Autodesk Fusion 360 part; units mm, degrees
note: some values were not read from the file. Chosen so that the rebuilt part matches the saved one: which bodies a step acts on; which face or edge a step refers to. Set by a fixed rule: which sketch regions a step uses.
(part 3 of 3)
sketch "Sketch30" plane through (0, 0, -52.6306) normal (0, 0, -1) x (1, 0, 0)
  line L0 (227.3311, -240.0788) -> (240.3311, -240.0788)
  line L1 (240.3311, -240.0788) -> (240.3311, -235.0788)
  line L2 (240.3311, -235.0788) -> (227.3311, -235.0788)
  line L3 (227.3311, -235.0788) -> (227.3311, -240.0788)
  line L4 (285, -250) -> (219.7748, -250)
  line L5 (219.7748, -250) -> (219.7748, 15.8116)
  line L6 (219.7748, 15.8116) -> (285, 15.8116)
  line L7 (285, 15.8116) -> (285, -250)
  line L8 (213.7748, -256) -> (213.7748, 21.8116)
  line L9 (213.7748, 21.8116) -> (291, 21.8116)
  line L10 (291, 21.8116) -> (291, -256)
  line L11 (291, -256) -> (213.7748, -256)
  dimension "d221" = -6
  constraint horizontal L4
  constraint vertical L5
  constraint horizontal L6
  constraint vertical L7
extrude "Extrude30" add sketch "Sketch30" against normal blind 25 separate body contours L0 L1 L2 L3 | L4 L5 L6 L7 | L8 L9 L10 L11 makes body 58
ref_plane "WorkPlane6" through (252.3874, 117.0942, -40.1306) normal (-1, 0, 0) x (0, -1, 0)
combine "Combine5" operation cut target body 58 tool bodies 39 keep tools
move_body "Move20" bodies 39 to x (1, 0, 0) y (0, 1, 0) z (0, 0, 1) at (-71.162, 94.4527, -197.0205)
split "Split5" by plane through (0, 0, -37.6306) normal (0, 0, -1) bodies 58 makes body 71 at (256.3686, -15.1815, -52.6306) makes body 64 at (270.9978, 2.7409, -44.9639) makes body 66 at (267.6644, 13.4167, -44.9639) makes body 68 at (270.9978, 38.0755, -41.2973) makes body 65 at (270.9978, 53.7409, -44.9639) makes body 63 at (270.9978, 70.7409, -44.9639) makes body 62 at (269.5811, 87.7409, -44.9639) makes body 62 at (269.5811, 138.6196, -45.2973) makes body 62 at (269.5811, 234.4167, -44.9639) makes body 60 at (235.0811, 149.4167, -44.9639) makes body 60 at (235.0811, 87.6196, -45.2973) makes body 60 at (235.0811, 2.7409, -44.9639) makes body 61 at (236.9978, 172.7409, -44.9639) makes body 70 at (233.6644, 189.7409, -44.9639) makes body 67 at (236.9978, 206.7409, -44.9639) makes body 59 at (236.9978, 223.7409, -44.9639) makes body 69 at (236.9978, 233.0822, -41.2973)
move_body "Move21" bodies 71 to x (1, 0, 0) y (0, 1, 0) z (0, 0, 1) at (-20.1654, 78.4525, -119.6361)
move_body "Move22" bodies 71 to x (1, 0, 0) y (0, 1, 0) z (0, 0, 1) at (167.4091, 25.7821, -64.3844)
move_body "Move23" bodies 39 to x (1, 0, 0) y (0, 1, 0) z (0, 0, 1) at (307.5343, 23.4357, 0)
combine "Combine6" operation add target body 59 tool bodies 58 62 61 63 65 64 60 67 68 66 69 70
sketch "Sketch33" plane through (0, 0, -234.6511) normal (0, 0, 1) x (-1, 0, 0)
  line L0 (-455.7033, -101.9673) -> (-521.7033, -101.9673)
  line L1 (-521.7033, -367.9673) -> (-455.7033, -367.9673)
  line L2 (-465.7033, -112.9673) -> (-465.7033, -357.9673)
  line L3 (-465.7033, -357.9673) -> (-511.7033, -357.9673)
  line L4 (-511.7033, -357.9673) -> (-511.7033, -112.9673)
  line L5 (-511.7033, -112.9673) -> (-465.7033, -112.9673)
  line L6 (-521.7033, -101.9673) -> (-521.7033, -367.9673)
  line L7 (-455.7033, -367.9673) -> (-455.7033, -101.9673)
  line L8 (-521.8033, -368.0673) -> (-455.6033, -368.0673)
  line L9 (-455.6033, -368.0673) -> (-455.6033, -101.8673)
  line L10 (-455.6033, -101.8673) -> (-521.8033, -101.8673)
  line L11 (-521.8033, -101.8673) -> (-521.8033, -368.0673)
extrude "Extrude31" add sketch "Sketch33" along normal blind 3.5 separate body contours L0 L1 L6 L7 | L2 L3 L4 L5 makes body 72
move_body "Move24" bodies 72 to x (1, 0, 0) y (0, 1, 0) z (0, 0, 1) at (-5.1974, -2.7632, 46.1585)
sketch "Sketch34" plane through (0, 0, -184.9926) normal (0, 0, 1) x (-1, 0, 0)
  line L0 (-450.5059, -99.2041) -> (-516.5059, -99.2041)
  line L1 (-516.5059, -365.2041) -> (-450.5059, -365.2041)
  line L2 (-530.7033, -90) -> (-439.8083, -90)
  line L3 (-439.8083, -90) -> (-439.8083, -380)
  line L4 (-439.8083, -380) -> (-530.7033, -380)
  line L5 (-530.7033, -380) -> (-530.7033, -90)
  line L6 (-513.7033, -175.6989) -> (-513.7033, -161.2357)
  line L7 (-450.5059, -365.2041) -> (-450.5059, -99.2041)
  line L8 (-516.5059, -99.2041) -> (-516.5059, -365.2041)
  dimension "d228" = 290
  dimension "d229" = 17
  constraint horizontal L2
  constraint vertical L3
  constraint horizontal L4
  constraint vertical L5
  measures "d228" distance of L2.start L4.end
  measures "d229" distance of L5 L6
extrude "Extrude32" add sketch "Sketch34" against normal blind 8 separate body contours L0 L1 L7 L8 | L2 L3 L4 L5 makes body 73
combine "Combine7" operation cut target body 73 tool bodies 72 keep tools
move_body "Move25" bodies 72 to x (1, 0, 0) y (0, 1, 0) z (0, 0, 1) at (-138.6238, -0.1199, 15.5638)
move_body "Move26" bodies 72 to x (1, 0, 0) y (0, 1, 0) z (0, 0, 1) at (143.8212, 2.8832, -61.7223)
move_body "Move27" bodies 73 to x (1, 0, 0) y (0, 1, 0) z (0, 0, 1) at (-72.8872, -94.5408, 54.1624)
move_body "Move28" bodies 71 to x (1, 0, 0) y (0, 1, 0) z (0, 0, 1) at (-18.7998, -23.1171, 16.5603)
move_body "Move29" bodies 72 to x (1, 0, 0) y (0, 1, 0) z (0, 0, 1) at (192.8594, 40.5329, 4.3772)
move_body "Move30" bodies 59 to x (1, 0, 0) y (0, -1, 0) z (0, 0, -1) at (0, 267.3186, -55.2612)
sketch "Sketch35" plane through (0, 0, -234.6511) normal (0, 0, 1) x (-1, 0, 0)
  line L0 (-521.7033, -101.9673) -> (-521.7033, -367.9673)
  line L1 (-521.7033, -367.9673) -> (-455.7033, -367.9673)
  line L2 (-455.7033, -367.9673) -> (-455.7033, -101.9673)
  line L3 (-455.7033, -101.9673) -> (-521.7033, -101.9673)
  line L4 (-465.7033, -112.9673) -> (-465.7033, -357.9673)
  line L5 (-465.7033, -357.9673) -> (-511.7033, -357.9673)
  line L6 (-511.7033, -357.9673) -> (-511.7033, -112.9673)
  line L7 (-511.7033, -112.9673) -> (-465.7033, -112.9673)
  line L8 (-521.7033, -367.9673) -> (-505.7033, -367.9673)
  line L9 (-505.7033, -353.9673) -> (-505.7033, -367.9673)
  line L10 (-455.7033, -367.9673) -> (-471.7033, -367.9673)
  line L11 (-471.7033, -367.9673) -> (-471.7033, -271.9673)
  dimension "d232" = 16
  dimension "d233" = 14
  dimension "d234" = 16
  dimension "d235" = 96
  constraint coincident L0.end L1.start
  constraint coincident L1 L8.end
  constraint perpendicular L0 L8
  constraint perpendicular L8 L9
  constraint coincident L1.end L2.start
  constraint coincident L1 L10.end
  constraint perpendicular L2 L10
  constraint perpendicular L10 L11
  measures "d232" distance of L0.end L8.end
  measures "d233" distance of L8.end L9.start
  measures "d234" distance of L1.end L10.end
  measures "d235" distance of L10.end L11.end
sketch "Sketch36" plane through (0, 0, -134.3303) normal (0, 0, 1) x (-1, 0, 0)
  line L0 (-377.6187, -270.6633) -> (-377.6187, -4.6633)
  line L1 (-377.6187, -4.6633) -> (-443.6187, -4.6633)
  line L2 (-443.6187, -4.6633) -> (-443.6187, -270.6633)
  line L3 (-443.6187, -270.6633) -> (-377.6187, -270.6633)
  line L4 (-443.6187, -270.6633) -> (-427.6187, -270.6633)
  line L5 (-377.6187, -270.6633) -> (-393.6187, -270.6633)
  line L6 (-427.6187, -270.6633) -> (-427.6187, -256.6633)
  line L7 (-393.6187, -270.6633) -> (-393.6187, -174.6633)
  circle A0 centre (-393.6187, -174.6633) radius 1
  circle A1 centre (-427.6187, -256.6633) radius 1
  dimension "d236" = 16
  dimension "d237" = 16
  dimension "d238" = 14
  dimension "d239" = 96
  dimension "d240" = 2
  dimension "d241" = 2
  constraint coincident L2.end L3.start
  constraint coincident L3 L4.end
  constraint perpendicular L2 L4
  constraint coincident L0.start L3.end
  constraint coincident L3 L5.end
  constraint perpendicular L0 L5
  constraint perpendicular L4 L6
  constraint perpendicular L5 L7
  constraint coincident L7.end A0.centre
  constraint coincident L6.end A1.centre
  measures "d236" distance of L2.end L4.end
  measures "d237" distance of L0.start L5.end
  measures "d238" distance of L4.end L6.end
  measures "d239" distance of L5.end L7.end
  measures "d240" diameter of A0
  measures "d241" diameter of A1
extrude "Extrude33" add sketch "Sketch36" along normal up to surface (3.5 mm away) contours A0 | A1 bodies 73
move_body "Move16" [suppressed]
move_body "Move17" [suppressed]
move_body "Move18" [suppressed]
move_body "Move19" [suppressed]
split "Split4" [suppressed]
move_body "Move15" [suppressed]
component "Component" placed x (1, 0, 0) y (0, 1, 0) z (0, 0, 1) at (0, 0, 0)
hidden bodies 47 55
